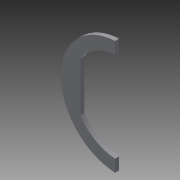
# Autodesk Inventor part: zablona_oblouk
Saved by Autodesk Inventor 2015 (Build 190159000, 159)
## iProperties
Created: 2015-01-02
Part Number: zablona_oblouk
Material: Generic
Document SubType Name: Modeling
Designer: Turboslimak
Density: 1 g/cm^3
Appearance: Default
Author: Turboslimak
Autodesk Inventor part; units mm, degrees
ref_plane "YZ Plane" through (0, 0, 0) normal (1, 0, 0) x (0, 1, 0)
ref_plane "XZ Plane" through (0, 0, 0) normal (0, 1, 0) x (-1, 0, 0)
ref_plane "XY Plane" through (0, 0, 0) normal (0, 0, 1) x (1, 0, 0)
sketch "Sketch1" plane through (0, 0, 0) normal (0, 1, 0) x (-1, 0, 0)
  line L0 (-32, 70.5) -> (-32, 55.5)
  line L1 (-32, -70.5) -> (-32, -55.5)
  arc A0 (11, 30.3335) -> (-32, 55.5) centre (-35.6178, 0) ccw
  arc A1 (-32, -55.5) -> (11, -30.3335) centre (-35.6178, 0) ccw
  line L2 (11, 30.3335) -> (11, -30.3335)
  arc A2 (-32, -70.5) -> (-32, 70.5) centre (-35.5914, 0) ccw
  line L3 (35, 0) -> (11, 0)
  point P0 (0, 0)
  dimension "d1" = 141
  dimension "d2" = 15
  dimension "d3" = 15
  dimension "d7" = 24
  constraints: 8 end point, 8 point on circle, 3 centre point, 1 midpoint, 1 vertical
  measures "d1" distance of L1.start L0.start
  measures "d2" distance of L0.start L0.end
  measures "d3" distance of L1.start L1.end
  measures "d7" distance of L3.start L3.end
extrude "Extrusion1" add sketch "Sketch1" along normal blind 5
body "Solid1"
